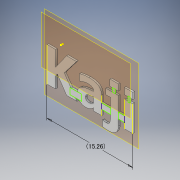
# Autodesk Inventor part: photon_sample
Saved by Autodesk Inventor 2019.3 (Build 233278000, 278)
## iProperties
Created: 2019-10-25
Part Number: photon_sample
Material: Generic
Document SubType Name: Modeling
Designer: ushiyama
Density: 1 g/cm^3
Appearance: Default
Author: ushiyama
Autodesk Inventor part; units mm, degrees
ref_plane "YZ Plane" through (0, 0, 0) normal (1, 0, 0) x (0, 1, 0)
ref_plane "XZ Plane" through (0, 0, 0) normal (0, 1, 0) x (-1, 0, 0)
sketch "スケッチ1" plane through (0, 0, 0) normal (0, 0, 1) x (1, 0, 0)
  line L0 (-3.1348, -0.9098) -> (10.2725, -0.9098) construction
  line L1 (10.2725, -0.9098) -> (10.2725, -4.9582) construction
  line L2 (10.2725, -4.9582) -> (-3.1348, -4.9582) construction
  line L3 (-3.1348, -4.9582) -> (-3.1348, -0.9098) construction
  line L4 (2.8417, -7.2866) -> (0.9879, -7.2866)
  line L5 (0.9879, -7.2866) -> (-0.6681, -4.8101)
  line L6 (-0.6681, -4.8101) -> (-0.9696, -5.2253)
  line L7 (-0.9696, -5.2253) -> (-0.9696, -7.2866)
  line L8 (-0.9696, -7.2866) -> (-2.502, -7.2866)
  line L9 (-2.502, -7.2866) -> (-2.502, -1.1866)
  line L10 (-2.502, -1.1866) -> (-0.9696, -1.1866)
  line L11 (-0.9696, -1.1866) -> (-0.9696, -3.9104)
  line L12 (-0.9696, -3.9104) -> (0.9879, -1.1866)
  line L13 (0.9879, -1.1866) -> (2.7527, -1.1866)
  line L14 (2.7527, -1.1866) -> (0.5776, -4.0191)
  line L15 (0.5776, -4.0191) -> (2.8417, -7.2866)
  spline S0 degree 2 poles (5.7928, -6.7973) (5.6445, -6.9208) (5.4122, -7.1186) (5.2144, -7.2174) knots 0 0 0 1 2 2 2
  spline S1 degree 2 poles (5.2144, -7.2174) (5.0216, -7.3114) (4.6558, -7.4102) (4.3296, -7.4102) knots 0 0 0 1 2 2 2
  spline S2 degree 2 poles (4.3296, -7.4102) (3.7166, -7.4102) (2.9109, -6.5896) (2.9109, -5.9668) knots 0 0 0 1 2 2 2
  spline S3 degree 2 poles (2.9109, -5.9668) (2.9109, -5.4576) (3.3212, -4.8249) (3.7067, -4.642) knots 0 0 0 1 2 2 2
  spline S4 degree 2 poles (3.7067, -4.642) (4.0973, -4.4542) (5.1798, -4.3059) (5.8027, -4.2663) knots 0 0 0 1 2 2 2
  line L16 (5.8027, -4.2663) -> (5.8027, -4.2416)
  spline S5 degree 2 poles (5.8027, -4.2416) (5.8027, -3.861) (5.2392, -3.5693) (4.6756, -3.5693) knots 0 0 0 1 2 2 2
  spline S6 degree 2 poles (4.6756, -3.5693) (4.4235, -3.5693) (3.7413, -3.7522) (3.42, -3.8956) knots 0 0 0 1 2 2 2
  line L17 (3.42, -3.8956) -> (3.2964, -3.8956)
  line L18 (3.2964, -3.8956) -> (3.2964, -2.7833)
  spline S7 degree 2 poles (3.2964, -2.7833) (3.509, -2.724) (4.4581, -2.5559) (4.9426, -2.5559) knots 0 0 0 1 2 2 2
  spline S8 degree 2 poles (4.9426, -2.5559) (6.1289, -2.5559) (7.2165, -3.3469) (7.2165, -4.1576) knots 0 0 0 1 2 2 2
  line L19 (7.2165, -4.1576) -> (7.2165, -7.2866)
  line L20 (7.2165, -7.2866) -> (5.7928, -7.2866)
  line L21 (5.7928, -7.2866) -> (5.7928, -6.7973)
  line L22 (5.7928, -6.0854) -> (5.7928, -5.1314)
  spline S9 degree 2 poles (5.7928, -5.1314) (5.427, -5.166) (4.9772, -5.2204) (4.7597, -5.2995) knots 0 0 0 1 2 2 2
  spline S10 degree 2 poles (4.7597, -5.2995) (4.5669, -5.3637) (4.3593, -5.6307) (4.3593, -5.8482) knots 0 0 0 1 2 2 2
  spline S11 degree 2 poles (4.3593, -5.8482) (4.3593, -6.1695) (4.7102, -6.4117) (5.0513, -6.4117) knots 0 0 0 1 2 2 2
  spline S12 degree 2 poles (5.0513, -6.4117) (5.2392, -6.4117) (5.6346, -6.2387) (5.7928, -6.0854) knots 0 0 0 1 2 2 2
  spline S13 degree 2 poles (10.2269, -7.3657) (10.2269, -8.1468) (9.3025, -9.0168) (8.5709, -9.0168) knots 0 0 0 1 2 2 2
  spline S14 degree 2 poles (8.5709, -9.0168) (8.1755, -9.0168) (7.5378, -8.9476) (7.3895, -8.908) knots 0 0 0 1 2 2 2
  line L23 (7.3895, -8.908) -> (7.3895, -7.8502)
  line L24 (7.3895, -7.8502) -> (7.4982, -7.8502)
  spline S15 degree 2 poles (7.4982, -7.8502) (7.6416, -7.8947) (7.9777, -7.949) (8.0815, -7.949) knots 0 0 0 1 2 2 2
  spline S16 degree 2 poles (8.0815, -7.949) (8.4968, -7.949) (8.7934, -7.4399) (8.7934, -6.8615) knots 0 0 0 1 2 2 2
  line L25 (8.7934, -6.8615) -> (8.7934, -3.683)
  line L26 (8.7934, -3.683) -> (7.9678, -3.683)
  line L27 (7.9678, -3.683) -> (7.9678, -2.6845)
  line L28 (7.9678, -2.6845) -> (10.2269, -2.6845)
  line L29 (10.2269, -2.6845) -> (10.2269, -7.3657)
  line L30 (10.2269, -2.027) -> (8.6994, -2.027)
  line L31 (8.6994, -2.027) -> (8.6994, -0.9098)
  line L32 (8.6994, -0.9098) -> (10.2269, -0.9098)
  line L33 (10.2269, -0.9098) -> (10.2269, -2.027)
  line L34 (12.7579, -7.2866) -> (11.3243, -7.2866)
  line L35 (11.3243, -7.2866) -> (11.3243, -2.6845)
  line L36 (11.3243, -2.6845) -> (12.7579, -2.6845)
  line L37 (12.7579, -2.6845) -> (12.7579, -7.2866)
  line L38 (12.8024, -2.027) -> (11.2848, -2.027)
  line L39 (11.2848, -2.027) -> (11.2848, -0.9098)
  line L40 (11.2848, -0.9098) -> (12.8024, -0.9098)
  line L41 (12.8024, -0.9098) -> (12.8024, -2.027)
  point P0 (0, 0)
  constraints: 2 other
extrude "押し出し1" add sketch "スケッチ1" along normal blind 0.3
ref_plane "作業平面1" through (0, 0, 0.3) normal (0, 0, 1) x (1, 0, 0)
sketch "スケッチ4" plane through (0, 0, 0.3) normal (0, 0, 1) x (1, 0, 0)
  line L0 (12.7579, -7.2866) -> (12.7579, -2.6845) projected
  line L1 (-2.502, -1.1866) -> (-2.502, -7.2866) projected
  line L2 (1.5924, -6.8642) -> (3.6217, -6.8642)
  line L3 (3.6217, -6.8642) -> (3.6217, -5.7481)
  line L4 (3.6217, -5.7481) -> (1.5924, -5.7481)
  line L5 (1.5924, -5.7481) -> (1.5924, -6.8642)
  line L6 (7.2165, -7.2866) -> (7.2165, -4.1576) projected
  line L7 (7.2165, -6.3062) -> (8.8066, -6.3062)
  line L8 (8.8066, -6.3062) -> (8.8066, -5.3089)
  line L9 (8.8066, -5.3089) -> (7.2165, -5.3089)
  line L10 (7.2165, -5.3089) -> (7.2165, -6.3062)
  line L11 (11.3243, -2.6845) -> (11.3243, -7.2866) projected
  line L12 (10.1491, -6.3062) -> (11.3243, -6.3062)
  line L13 (11.3243, -6.3062) -> (11.3243, -5.234)
  line L14 (11.3243, -5.234) -> (10.1491, -5.234)
  line L15 (10.1491, -5.234) -> (10.1491, -6.3062)
  line L16 (9.1301, -2.6845) -> (9.6378, -2.6845)
  line L17 (9.6378, -2.6845) -> (9.6378, -1.9909)
  line L18 (9.6378, -1.9909) -> (9.1301, -1.9909)
  line L19 (9.1301, -1.9909) -> (9.1301, -2.6845)
  line L20 (11.8767, -2.8267) -> (12.226, -2.8267)
  line L21 (12.226, -2.8267) -> (12.226, -1.8839)
  line L22 (12.226, -1.8839) -> (11.8767, -1.8839)
  line L23 (11.8767, -1.8839) -> (11.8767, -2.8267)
  point P0 (0, 0)
  dimension "d6" = 15.2599
  constraints: 40 end point, 10 parallel, 5 horizontal, 5 perpendicular, 3 point on line
  measures "d6" distance between parallel lines of L0 L1
extrude "押し出し3" add sketch "スケッチ4" against normal blind 0.3 contours L5 L4 L3 L2 | L6 L9 L8 L7 | L11 L12 L15 L14
extrude "押し出し4" add sketch "スケッチ4" against normal blind 0.3 contours L19 L18 L17 L16 | L23 L22 L21 L20
